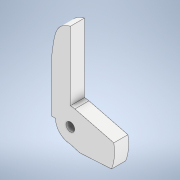
# Autodesk Inventor part: end_cap
Saved by Autodesk Inventor 2022 (Build 260153000, 153)
## iProperties
Created: 2022-12-27
Part Number: end_cap
Material: Типовые
Document SubType Name: Modeling
Designer: akapu
Density: 1 g/cm^3
Appearance: По умолчанию
Author: akapu
Autodesk Inventor part; units mm, degrees
ref_plane "YZ Plane" through (0, 0, 0) normal (1, 0, 0) x (0, 1, 0)
ref_plane "XZ Plane" through (0, 0, 0) normal (0, 1, 0) x (-1, 0, 0)
ref_plane "XY Plane" through (0, 0, 0) normal (0, 0, 1) x (1, 0, 0)
sketch "Эскиз1" plane through (0, 0, 0) normal (0, 0, 1) x (1, 0, 0)
  circle A0 centre (-7, -17) radius 1.5 projected
  line L0 (14, -14.4) -> (14, -5) projected
  arc A1 (14, -5) -> (11, -2) centre (11, -5) ccw projected
  line L1 (11, -2) -> (-7, -2) projected
  line L2 (-7, -2) -> (-7, 15) projected
  line L3 (-14, 9.5) -> (-14, -8.75) projected
  line L4 (-7, -24) -> (7, -24) projected
  arc A2 (7, -24) -> (13.4992, -14.4) centre (7, -17) ccw projected
  line L5 (13.4992, -14.4) -> (14, -14.4) projected
  circle A3 centre (7, -17) radius 2.5 projected
  circle A4 centre (-7, -8.75) radius 5.5 projected
  circle A5 centre (-7, -8.75) radius 6.75 projected
  circle A6 centre (-7, -8.75) radius 5.5 projected
  circle A7 centre (-7, -8.75) radius 16.2607 projected
  circle A8 centre (-7, -8.75) radius 6.75 projected
  circle A9 centre (-7, -8.75) radius 5.5 projected
  arc A10 (46.8183, -61.5099) -> (48.485, -59.5378) centre (46.485, -59.5378) ccw projected
  line L6 (48.485, -59.5378) -> (48.485, -18) projected
  arc A11 (51.485, -15) -> (48.485, -18) centre (51.485, -18) ccw projected
  line L7 (51.485, -15) -> (51.97, -15) projected
  arc A12 (51.97, -15) -> (54.97, -12) centre (51.97, -12) ccw projected
  line L8 (54.97, -5) -> (54.97, -12) projected
  arc A13 (54.97, -5) -> (51.97, -2) centre (51.97, -5) ccw projected
  line L9 (-0.3729, -2) -> (51.97, -2) projected
  arc A14 (-0.3729, -2) -> (-11.03, -11.2398) centre (-0.1714, -12.9982) ccw projected
  line L10 (-11.03, -11.2398) -> (-11.03, -20.501) projected
  arc A15 (-11.03, -20.501) -> (-9.8871, -23.3004) centre (-7.03, -20.501) ccw projected
  arc A16 (-9.03, -25.4) -> (-9.8871, -23.3004) centre (-12.03, -25.4) ccw projected
  line L11 (-9.03, -25.4) -> (-9.03, -104.6) projected
  arc A17 (-9.8871, -106.6996) -> (-9.03, -104.6) centre (-12.03, -104.6) ccw projected
  arc A18 (-9.8871, -106.6996) -> (-11.03, -109.499) centre (-7.03, -109.499) ccw projected
  line L12 (-11.03, -109.499) -> (-11.03, -118.7602) projected
  arc A19 (-11.03, -118.7602) -> (-0.3729, -128) centre (-0.1714, -117.0018) ccw projected
  line L13 (51.97, -128) -> (-0.3729, -128) projected
  arc A20 (51.97, -128) -> (54.97, -125) centre (51.97, -125) ccw projected
  line L14 (54.97, -118) -> (54.97, -125) projected
  arc A21 (54.97, -118) -> (51.97, -115) centre (51.97, -118) ccw projected
  line L15 (51.97, -115) -> (51.485, -115) projected
  arc A22 (48.485, -112) -> (51.485, -115) centre (51.485, -112) ccw projected
  line L16 (48.485, -112) -> (48.485, -80.5022) projected
  arc A23 (48.485, -80.5022) -> (46.8183, -78.5301) centre (46.485, -80.5022) ccw projected
  arc A24 (43.485, -77.3303) -> (46.8183, -78.5301) centre (48.485, -68.67) ccw projected
  arc A25 (42.485, -75.5982) -> (43.485, -77.3303) centre (44.485, -75.5982) ccw projected
  line L17 (42.485, -75.5982) -> (42.485, -64.4418) projected
  arc A26 (43.485, -62.7097) -> (42.485, -64.4418) centre (44.485, -64.4418) ccw projected
  arc A27 (46.8183, -61.5099) -> (43.485, -62.7097) centre (48.485, -71.37) ccw projected
  circle A28 centre (-7, -113) radius 1.5 projected
  circle A29 centre (-7, -17) radius 1.5 projected
  circle A30 centre (48.485, -121.515) radius 1.5 projected
  circle A31 centre (7, -83) radius 1.5 projected
  circle A32 centre (7, -47) radius 1.5 projected
  circle A33 centre (48.485, -8.485) radius 1.5 projected
  circle A34 centre (39.485, -9.27) radius 0.325 projected
  circle A35 centre (38.885, -57.77) radius 0.8 projected
  circle A36 centre (39.385, -64.52) radius 0.5 projected
  circle A37 centre (-5.73, -68.27) radius 0.325 projected
  circle A38 centre (18.2, -105.38) radius 0.325 projected
  circle A39 centre (2.77, -17) radius 0.325 projected
  circle A40 centre (45.185, -81.79) radius 0.325 projected
  circle A41 centre (45.185, -36.51) radius 0.325 projected
  circle A42 centre (2.77, -10) radius 0.325 projected
  circle A43 centre (2.77, -120) radius 0.325 projected
  circle A44 centre (-5.73, -55.42) radius 0.325 projected
  circle A45 centre (29.385, -72.52) radius 0.85 projected
  circle A46 centre (43.885, -57.77) radius 0.8 projected
  circle A47 centre (-1.23, -120) radius 0.325 projected
  circle A48 centre (29.385, -67.52) radius 0.85 projected
  circle A49 centre (18.2, -92.76) radius 0.325 projected
  circle A50 centre (-5.73, -79) radius 0.325 projected
  circle A51 centre (35.215, -122) radius 0.325 projected
  circle A52 centre (33.485, -7.27) radius 0.5 projected
  circle A53 centre (45.185, -101.03) radius 0.325 projected
  circle A54 centre (45.185, -16.27) radius 0.325 projected
  circle A55 centre (35.215, -115) radius 0.325 projected
  circle A56 centre (2.77, -113) radius 0.325 projected
  circle A57 centre (-5.73, -40.84) radius 0.325 projected
  circle A58 centre (39.385, -75.52) radius 0.5 projected
  circle A59 centre (-1.23, -10) radius 0.325 projected
  arc A60 (46.8183, -61.5099) -> (48.485, -59.5378) centre (46.485, -59.5378) ccw projected
  line L18 (48.485, -59.5378) -> (48.485, -18) projected
  arc A61 (51.485, -15) -> (48.485, -18) centre (51.485, -18) ccw projected
  line L19 (51.485, -15) -> (51.97, -15) projected
  arc A62 (51.97, -15) -> (54.97, -12) centre (51.97, -12) ccw projected
  line L20 (54.97, -5) -> (54.97, -12) projected
  arc A63 (54.97, -5) -> (51.97, -2) centre (51.97, -5) ccw projected
  line L21 (-0.3729, -2) -> (51.97, -2) projected
  arc A64 (-0.3729, -2) -> (-11.03, -11.2398) centre (-0.1714, -12.9982) ccw projected
  line L22 (-11.03, -11.2398) -> (-11.03, -20.501) projected
  arc A65 (-11.03, -20.501) -> (-9.8871, -23.3004) centre (-7.03, -20.501) ccw projected
  arc A66 (-9.03, -25.4) -> (-9.8871, -23.3004) centre (-12.03, -25.4) ccw projected
  line L23 (-9.03, -25.4) -> (-9.03, -104.6) projected
  arc A67 (-9.8871, -106.6996) -> (-9.03, -104.6) centre (-12.03, -104.6) ccw projected
  arc A68 (-9.8871, -106.6996) -> (-11.03, -109.499) centre (-7.03, -109.499) ccw projected
  line L24 (-11.03, -109.499) -> (-11.03, -118.7602) projected
  arc A69 (-11.03, -118.7602) -> (-0.3729, -128) centre (-0.1714, -117.0018) ccw projected
  line L25 (51.97, -128) -> (-0.3729, -128) projected
  arc A70 (51.97, -128) -> (54.97, -125) centre (51.97, -125) ccw projected
  line L26 (54.97, -118) -> (54.97, -125) projected
  arc A71 (54.97, -118) -> (51.97, -115) centre (51.97, -118) ccw projected
  line L27 (51.97, -115) -> (51.485, -115) projected
  arc A72 (48.485, -112) -> (51.485, -115) centre (51.485, -112) ccw projected
  line L28 (48.485, -112) -> (48.485, -80.5022) projected
  arc A73 (48.485, -80.5022) -> (46.8183, -78.5301) centre (46.485, -80.5022) ccw projected
  arc A74 (43.485, -77.3303) -> (46.8183, -78.5301) centre (48.485, -68.67) ccw projected
  arc A75 (42.485, -75.5982) -> (43.485, -77.3303) centre (44.485, -75.5982) ccw projected
  line L29 (42.485, -75.5982) -> (42.485, -64.4418) projected
  arc A76 (43.485, -62.7097) -> (42.485, -64.4418) centre (44.485, -64.4418) ccw projected
  arc A77 (46.8183, -61.5099) -> (43.485, -62.7097) centre (48.485, -71.37) ccw projected
  circle A78 centre (-7, -113) radius 1.5 projected
  circle A79 centre (-7, -17) radius 1.5 projected
  circle A80 centre (48.485, -121.515) radius 1.5 projected
  circle A81 centre (7, -83) radius 1.5 projected
  circle A82 centre (7, -47) radius 1.5 projected
  circle A83 centre (48.485, -8.485) radius 1.5 projected
  circle A84 centre (39.485, -9.27) radius 0.325 projected
  circle A85 centre (38.885, -57.77) radius 0.8 projected
  circle A86 centre (39.385, -64.52) radius 0.5 projected
  circle A87 centre (-5.73, -68.27) radius 0.325 projected
  circle A88 centre (18.2, -105.38) radius 0.325 projected
  circle A89 centre (2.77, -17) radius 0.325 projected
  circle A90 centre (45.185, -81.79) radius 0.325 projected
  circle A91 centre (45.185, -36.51) radius 0.325 projected
  circle A92 centre (2.77, -10) radius 0.325 projected
  circle A93 centre (2.77, -120) radius 0.325 projected
  circle A94 centre (-5.73, -55.42) radius 0.325 projected
  circle A95 centre (29.385, -72.52) radius 0.85 projected
  circle A96 centre (43.885, -57.77) radius 0.8 projected
  circle A97 centre (-1.23, -120) radius 0.325 projected
  circle A98 centre (29.385, -67.52) radius 0.85 projected
  circle A99 centre (18.2, -92.76) radius 0.325 projected
  circle A100 centre (-5.73, -79) radius 0.325 projected
  circle A101 centre (35.215, -122) radius 0.325 projected
  circle A102 centre (33.485, -7.27) radius 0.5 projected
  circle A103 centre (45.185, -101.03) radius 0.325 projected
  circle A104 centre (45.185, -16.27) radius 0.325 projected
  circle A105 centre (35.215, -115) radius 0.325 projected
  circle A106 centre (2.77, -113) radius 0.325 projected
  circle A107 centre (-5.73, -40.84) radius 0.325 projected
  circle A108 centre (39.385, -75.52) radius 0.5 projected
  circle A109 centre (-1.23, -10) radius 0.325 projected
  circle A110 centre (-7, -17) radius 1.5 projected
  circle A111 centre (7, -17) radius 2.5 projected
  circle A112 centre (-7, -8.75) radius 16.2607 projected
  arc A113 (46.8183, -61.5099) -> (48.485, -59.5378) centre (46.485, -59.5378) ccw projected
  line L30 (48.485, -59.5378) -> (48.485, -18) projected
  arc A114 (51.485, -15) -> (48.485, -18) centre (51.485, -18) ccw projected
  line L31 (51.485, -15) -> (51.97, -15) projected
  arc A115 (51.97, -15) -> (54.97, -12) centre (51.97, -12) ccw projected
  line L32 (54.97, -5) -> (54.97, -12) projected
  arc A116 (54.97, -5) -> (51.97, -2) centre (51.97, -5) ccw projected
  line L33 (-0.3729, -2) -> (51.97, -2) projected
  arc A117 (-0.3729, -2) -> (-11.03, -11.2398) centre (-0.1714, -12.9982) ccw projected
  line L34 (-11.03, -11.2398) -> (-11.03, -20.501) projected
  arc A118 (-11.03, -20.501) -> (-9.8871, -23.3004) centre (-7.03, -20.501) ccw projected
  arc A119 (-9.03, -25.4) -> (-9.8871, -23.3004) centre (-12.03, -25.4) ccw projected
  line L35 (-9.03, -25.4) -> (-9.03, -104.6) projected
  arc A120 (-9.8871, -106.6996) -> (-9.03, -104.6) centre (-12.03, -104.6) ccw projected
  arc A121 (-9.8871, -106.6996) -> (-11.03, -109.499) centre (-7.03, -109.499) ccw projected
  line L36 (-11.03, -109.499) -> (-11.03, -118.7602) projected
  arc A122 (-11.03, -118.7602) -> (-0.3729, -128) centre (-0.1714, -117.0018) ccw projected
  line L37 (51.97, -128) -> (-0.3729, -128) projected
  arc A123 (51.97, -128) -> (54.97, -125) centre (51.97, -125) ccw projected
  line L38 (54.97, -118) -> (54.97, -125) projected
  arc A124 (54.97, -118) -> (51.97, -115) centre (51.97, -118) ccw projected
  line L39 (51.97, -115) -> (51.485, -115) projected
  arc A125 (48.485, -112) -> (51.485, -115) centre (51.485, -112) ccw projected
  line L40 (48.485, -112) -> (48.485, -80.5022) projected
  arc A126 (48.485, -80.5022) -> (46.8183, -78.5301) centre (46.485, -80.5022) ccw projected
  arc A127 (43.485, -77.3303) -> (46.8183, -78.5301) centre (48.485, -68.67) ccw projected
  arc A128 (42.485, -75.5982) -> (43.485, -77.3303) centre (44.485, -75.5982) ccw projected
  line L41 (42.485, -75.5982) -> (42.485, -64.4418) projected
  arc A129 (43.485, -62.7097) -> (42.485, -64.4418) centre (44.485, -64.4418) ccw projected
  arc A130 (46.8183, -61.5099) -> (43.485, -62.7097) centre (48.485, -71.37) ccw projected
  circle A131 centre (-7, -113) radius 1.5 projected
  circle A132 centre (-7, -17) radius 1.5 projected
  circle A133 centre (48.485, -121.515) radius 1.5 projected
  circle A134 centre (7, -83) radius 1.5 projected
  circle A135 centre (7, -47) radius 1.5 projected
  circle A136 centre (48.485, -8.485) radius 1.5 projected
  circle A137 centre (39.485, -9.27) radius 0.325 projected
  circle A138 centre (38.885, -57.77) radius 0.8 projected
  circle A139 centre (39.385, -64.52) radius 0.5 projected
  circle A140 centre (-5.73, -68.27) radius 0.325 projected
  circle A141 centre (18.2, -105.38) radius 0.325 projected
  circle A142 centre (2.77, -17) radius 0.325 projected
  circle A143 centre (45.185, -81.79) radius 0.325 projected
  circle A144 centre (45.185, -36.51) radius 0.325 projected
  circle A145 centre (2.77, -10) radius 0.325 projected
  circle A146 centre (2.77, -120) radius 0.325 projected
  circle A147 centre (-5.73, -55.42) radius 0.325 projected
  circle A148 centre (29.385, -72.52) radius 0.85 projected
  circle A149 centre (43.885, -57.77) radius 0.8 projected
  circle A150 centre (-1.23, -120) radius 0.325 projected
  circle A151 centre (29.385, -67.52) radius 0.85 projected
  circle A152 centre (18.2, -92.76) radius 0.325 projected
  circle A153 centre (-5.73, -79) radius 0.325 projected
  circle A154 centre (35.215, -122) radius 0.325 projected
  circle A155 centre (33.485, -7.27) radius 0.5 projected
  circle A156 centre (45.185, -101.03) radius 0.325 projected
  circle A157 centre (45.185, -16.27) radius 0.325 projected
  circle A158 centre (35.215, -115) radius 0.325 projected
  circle A159 centre (2.77, -113) radius 0.325 projected
  circle A160 centre (-5.73, -40.84) radius 0.325 projected
  circle A161 centre (39.385, -75.52) radius 0.5 projected
  circle A162 centre (-1.23, -10) radius 0.325 projected
  line L42 (-3.5, -15.3) -> (8.172, -14.6) projected
  line L43 (-1.9964, -14.2379) -> (9.1448, -10.6884) projected
  line L44 (7.4875, -11.5) -> (-3.5, -15.5) projected
  line L45 (-3.5, -15.3) -> (8.172, -14.6) projected
  line L46 (8.172, -14.8) -> (-3.5, -15.5) projected
  arc A163 (8.1929, -15.5) -> (7.4875, -11.5) centre (-3.5, -15.5) ccw projected
  line L47 (-3.5, -15.5) -> (9.3, -15.5) projected
  line L48 (-3.5, -15.5) -> (9.3, -15.5) projected
  circle A164 centre (-7, -17) radius 1.5 projected
  line L49 (14, -14.4) -> (14, -5) projected
  arc A165 (14, -5) -> (11, -2) centre (11, -5) ccw projected
  line L50 (11, -2) -> (-7, -2) projected
  line L51 (-7, -2) -> (-7, 15) projected
  line L52 (-14, 9.5) -> (-14, -8.75) projected
  line L53 (-7, -24) -> (7, -24) projected
  arc A166 (7, -24) -> (13.4992, -14.4) centre (7, -17) ccw projected
  line L54 (13.4992, -14.4) -> (14, -14.4) projected
  circle A167 centre (7, -17) radius 2.5 projected
  circle A168 centre (-7, -17) radius 1.5 projected
  line L55 (14, -14.4) -> (14, -5) projected
  arc A169 (14, -5) -> (11, -2) centre (11, -5) ccw projected
  line L56 (11, -2) -> (-7, -2) projected
  line L57 (-7, -2) -> (-7, 15) projected
  line L58 (-14, 9.5) -> (-14, -8.75) projected
  line L59 (-7, -24) -> (7, -24) projected
  arc A170 (7, -24) -> (13.4992, -14.4) centre (7, -17) ccw projected
  line L60 (13.4992, -14.4) -> (14, -14.4) projected
  circle A171 centre (7, -17) radius 2.5 projected
  line L61 (-3.5, -25.6) -> (-3.5, -15.5) projected
  line L62 (-3.5, -25.6) -> (-3.5, -15.5) projected
  line L63 (-3.5, -15.3) -> (-6.2824, -14.501) projected
  circle A172 centre (-7, -17) radius 2.6 projected
  line L64 (-3.5, -15.5) -> (-7, -15.5) projected
  circle A173 centre (-7, -17) radius 1.5 projected
  line L65 (14, -14.4) -> (14, -5) projected
  arc A174 (14, -5) -> (11, -2) centre (11, -5) ccw projected
  line L66 (11, -2) -> (-7, -2) projected
  line L67 (-7, -2) -> (-7, 15) projected
  line L68 (-14, 9.5) -> (-14, -8.75) projected
  line L69 (-7, -24) -> (7, -24) projected
  arc A175 (7, -24) -> (13.4992, -14.4) centre (7, -17) ccw projected
  line L70 (13.4992, -14.4) -> (14, -14.4) projected
  circle A176 centre (7, -17) radius 2.5 projected
  circle A177 centre (-7, -17) radius 1.5 projected
  circle A178 centre (-7, -17) radius 2.6 projected
  circle A179 centre (-7, -8.75) radius 5.5 projected
  line L71 (-1.9964, -14.2379) -> (-4.8898, -14.1478) projected
  line L72 (-1.9964, -14.2379) -> (9.1448, -10.6884) projected
  line L73 (-1.9964, -14.2379) -> (9.1448, -10.6884) projected
  circle A180 centre (-7, -8.75) radius 6.75 projected
  line L74 (-5.8077, -14.1192) -> (-4.8898, -14.1478) projected
  line L75 (-5.8077, -14.1192) -> (-4.8898, -14.1478) projected
  circle A181 centre (-7, -8.75) radius 5.5 projected
  line L76 (-7, -15.5) -> (-7, -2) projected
  line L77 (-7.1651, -14.2475) -> (-6.2824, -14.501) projected
  line L78 (-3.5, -15.3) -> (-6.2824, -14.501) projected
  circle A182 centre (-7, -17) radius 1.5 projected
  line L79 (14, -14.4) -> (14, -5) projected
  arc A183 (14, -5) -> (11, -2) centre (11, -5) ccw projected
  line L80 (11, -2) -> (-7, -2) projected
  line L81 (-7, -2) -> (-7, 15) projected
  line L82 (-14, 9.5) -> (-14, -8.75) projected
  line L83 (-7, -24) -> (7, -24) projected
  arc A184 (7, -24) -> (13.4992, -14.4) centre (7, -17) ccw projected
  line L84 (13.4992, -14.4) -> (14, -14.4) projected
  circle A185 centre (7, -17) radius 2.5 projected
  circle A186 centre (-7, -17) radius 2.6 projected
  circle A187 centre (-7, -17) radius 2.6 projected
  line L85 (-7, -15.5) -> (-7, -2) projected
  circle A188 centre (-7, -17) radius 1.5 projected
  line L86 (14, -14.4) -> (14, -5) projected
  arc A189 (14, -5) -> (11, -2) centre (11, -5) ccw projected
  line L87 (11, -2) -> (-7, -2) projected
  line L88 (-7, -2) -> (-7, 15) projected
  line L89 (-14, 9.5) -> (-14, -8.75) projected
  line L90 (-7, -24) -> (7, -24) projected
  arc A190 (7, -24) -> (13.4992, -14.4) centre (7, -17) ccw projected
  line L91 (13.4992, -14.4) -> (14, -14.4) projected
  circle A191 centre (7, -17) radius 2.5 projected
  circle A192 centre (-7, -17) radius 1.5 projected
  line L92 (14, -14.4) -> (14, -5) projected
  arc A193 (14, -5) -> (11, -2) centre (11, -5) ccw projected
  line L93 (11, -2) -> (-7, -2) projected
  line L94 (-7, -2) -> (-7, 15) projected
  line L95 (-14, 9.5) -> (-14, -8.75) projected
  line L96 (-7, -24) -> (7, -24) projected
  arc A194 (7, -24) -> (13.4992, -14.4) centre (7, -17) ccw projected
  line L97 (13.4992, -14.4) -> (14, -14.4) projected
  circle A195 centre (7, -17) radius 2.5 projected
  circle A196 centre (-7, -8.75) radius 5.5 projected
  circle A197 centre (-7, -17) radius 1.5 projected
  line L98 (14, -14.4) -> (14, -5) projected
  arc A198 (14, -5) -> (11, -2) centre (11, -5) ccw projected
  line L99 (11, -2) -> (-7, -2) projected
  line L100 (-7, -2) -> (-7, 15) projected
  line L101 (-14, 9.5) -> (-14, -8.75) projected
  line L102 (-7, -24) -> (7, -24) projected
  arc A199 (7, -24) -> (13.4992, -14.4) centre (7, -17) ccw projected
  line L103 (13.4992, -14.4) -> (14, -14.4) projected
  circle A200 centre (7, -17) radius 2.5 projected
  circle A201 centre (-7, -8.75) radius 1.6 projected
  circle A202 centre (-7, -8.75) radius 1.6 projected
  line L104 (-7, -15.5) -> (-7, -2) projected
  circle A203 centre (-7, -17) radius 1.5 projected
  line L105 (14, -14.4) -> (14, -5) projected
  arc A204 (14, -5) -> (11, -2) centre (11, -5) ccw projected
  line L106 (11, -2) -> (-7, -2) projected
  line L107 (-7, -2) -> (-7, 15) projected
  line L108 (-14, 9.5) -> (-14, -8.75) projected
  line L109 (-7, -24) -> (7, -24) projected
  arc A205 (7, -24) -> (13.4992, -14.4) centre (7, -17) ccw projected
  line L110 (13.4992, -14.4) -> (14, -14.4) projected
  circle A206 centre (7, -17) radius 2.5 projected
  circle A207 centre (-7, -17) radius 1.5 projected
  line L111 (14, -14.4) -> (14, -5) projected
  arc A208 (14, -5) -> (11, -2) centre (11, -5) ccw projected
  line L112 (11, -2) -> (-7, -2) projected
  line L113 (-7, -2) -> (-7, 15) projected
  line L114 (-14, 9.5) -> (-14, -8.75) projected
  line L115 (-7, -24) -> (7, -24) projected
  arc A209 (7, -24) -> (13.4992, -14.4) centre (7, -17) ccw projected
  line L116 (13.4992, -14.4) -> (14, -14.4) projected
  circle A210 centre (7, -17) radius 2.5 projected
  line L117 (-7, -8.75) -> (8.9993, -5.8462) projected
  circle A211 centre (-7, -17) radius 1.5 projected
  line L118 (14, -14.4) -> (14, -5) projected
  arc A212 (14, -5) -> (11, -2) centre (11, -5) ccw projected
  line L119 (11, -2) -> (-7, -2) projected
  line L120 (-7, -2) -> (-7, 15) projected
  line L121 (-14, 9.5) -> (-14, -8.75) projected
  line L122 (-7, -24) -> (7, -24) projected
  arc A213 (7, -24) -> (13.4992, -14.4) centre (7, -17) ccw projected
  line L123 (13.4992, -14.4) -> (14, -14.4) projected
  circle A214 centre (7, -17) radius 2.5 projected
  line L124 (7.7935, -2) -> (-7, -8.75) projected
  line L125 (7.7935, -2) -> (-7, -8.75) projected
  circle A215 centre (-7, -17) radius 1.5 projected
  line L126 (14, -14.4) -> (14, -5) projected
  arc A216 (14, -5) -> (11, -2) centre (11, -5) ccw projected
  line L127 (11, -2) -> (-7, -2) projected
  line L128 (-7, -2) -> (-7, 15) projected
  line L129 (-14, 9.5) -> (-14, -8.75) projected
  line L130 (-7, -24) -> (7, -24) projected
  arc A217 (7, -24) -> (13.4992, -14.4) centre (7, -17) ccw projected
  line L131 (13.4992, -14.4) -> (14, -14.4) projected
  circle A218 centre (7, -17) radius 2.5 projected
  circle A219 centre (-7, -8.75) radius 6.75 projected
  circle A220 centre (-7, -17) radius 1.5 projected
  line L132 (14, -14.4) -> (14, -5) projected
  arc A221 (14, -5) -> (11, -2) centre (11, -5) ccw projected
  line L133 (11, -2) -> (-7, -2) projected
  line L134 (-7, -2) -> (-7, 15) projected
  line L135 (-14, 9.5) -> (-14, -8.75) projected
  line L136 (-7, -24) -> (7, -24) projected
  arc A222 (7, -24) -> (13.4992, -14.4) centre (7, -17) ccw projected
  line L137 (13.4992, -14.4) -> (14, -14.4) projected
  circle A223 centre (7, -17) radius 2.5 projected
  circle A224 centre (-7, -8.75) radius 6.75 projected
  circle A225 centre (-7, -17) radius 2.6 projected
  circle A226 centre (-7, -17) radius 2.6 projected
  circle A227 centre (-7, -17) radius 1.5 projected
  line L138 (14, -14.4) -> (14, -5) projected
  arc A228 (14, -5) -> (11, -2) centre (11, -5) ccw projected
  line L139 (11, -2) -> (-7, -2) projected
  line L140 (-7, -2) -> (-7, 15) projected
  line L141 (-14, 9.5) -> (-14, -8.75) projected
  line L142 (-7, -24) -> (7, -24) projected
  arc A229 (7, -24) -> (13.4992, -14.4) centre (7, -17) ccw projected
  line L143 (13.4992, -14.4) -> (14, -14.4) projected
  circle A230 centre (7, -17) radius 2.5 projected
  line L144 (8.9993, -5.8462) -> (-1.6265, -3.1497) projected
  line L145 (8.9993, -5.8462) -> (-1.6265, -3.1497) projected
  circle A231 centre (-7, -17) radius 1.5 projected
  line L146 (14, -14.4) -> (14, -5) projected
  arc A232 (14, -5) -> (11, -2) centre (11, -5) ccw projected
  line L147 (11, -2) -> (-7, -2) projected
  line L148 (-7, -2) -> (-7, 15) projected
  line L149 (-14, 9.5) -> (-14, -8.75) projected
  line L150 (-7, -24) -> (7, -24) projected
  arc A233 (7, -24) -> (13.4992, -14.4) centre (7, -17) ccw projected
  line L151 (13.4992, -14.4) -> (14, -14.4) projected
  circle A234 centre (7, -17) radius 2.5 projected
  circle A235 centre (-7, -17) radius 1.5 projected
  line L152 (14, -14.4) -> (14, -5) projected
  arc A236 (14, -5) -> (11, -2) centre (11, -5) ccw projected
  line L153 (11, -2) -> (-7, -2) projected
  line L154 (-7, -2) -> (-7, 15) projected
  line L155 (-14, 9.5) -> (-14, -8.75) projected
  line L156 (-7, -24) -> (7, -24) projected
  arc A237 (7, -24) -> (13.4992, -14.4) centre (7, -17) ccw projected
  line L157 (13.4992, -14.4) -> (14, -14.4) projected
  circle A238 centre (7, -17) radius 2.5 projected
  circle A239 centre (-7, -17) radius 1.5 projected
  line L158 (14, -14.4) -> (14, -5) projected
  arc A240 (14, -5) -> (11, -2) centre (11, -5) ccw projected
  line L159 (11, -2) -> (-7, -2) projected
  line L160 (-7, -2) -> (-7, 15) projected
  line L161 (-14, 9.5) -> (-14, -8.75) projected
  line L162 (-7, -24) -> (7, -24) projected
  arc A241 (7, -24) -> (13.4992, -14.4) centre (7, -17) ccw projected
  line L163 (13.4992, -14.4) -> (14, -14.4) projected
  circle A242 centre (7, -17) radius 2.5 projected
  circle A243 centre (-7, -8.75) radius 6.75 projected
  line L164 (11, -2) -> (-7, -2) projected
  circle A244 centre (-7, -17) radius 1.5 projected
  line L165 (14, -14.4) -> (14, -5) projected
  arc A245 (14, -5) -> (11, -2) centre (11, -5) ccw projected
  line L166 (11, -2) -> (-7, -2) projected
  line L167 (-7, -2) -> (-7, 15) projected
  line L168 (-14, 9.5) -> (-14, -8.75) projected
  line L169 (-7, -24) -> (7, -24) projected
  arc A246 (7, -24) -> (13.4992, -14.4) centre (7, -17) ccw projected
  line L170 (13.4992, -14.4) -> (14, -14.4) projected
  circle A247 centre (7, -17) radius 2.5 projected
  line L171 (-7, 15) -> (-7, 23.3611) projected
  line L172 (8.9993, -5.8462) -> (-1.6265, -3.1497) projected
  line L173 (8.9993, -5.8462) -> (-6.1569, -2) projected
  line L174 (8.9993, -5.8462) -> (-1.6265, -3.1497) projected
  line L175 (8.9993, -5.8462) -> (-6.1569, -2) projected
  line L176 (-14, -8.75) -> (-14, -3.75)
  line L177 (-14, -8.75) -> (-12.5, -8.75)
  spline S0 degree 3 poles (-7, 23.3611) (-12.8051, 21.7936) (-12.8999, 17.7118) (-14, 9.5) knots -0.659309 -0.659309 -0.659309 -0.659309 0 0 0 0 projected
  line L178 (-14, -8.75) -> (-12.7, -8.75) projected
  arc A248 (-12.7, -8.75) -> (-11.9767, -11.529) centre (-7, -8.75) ccw projected
  line L179 (-11.9767, -11.529) -> (-9.4156, -17.9617) projected
  arc A249 (-9.4156, -17.9617) -> (-7, -19.6) centre (-7, -17) ccw projected
  arc A250 (-7, -24) -> (-7, -19.6) centre (-7, -21.8) ccw projected
  line L180 (-7, 15) -> (-7, 23.3611) projected
  spline S1 degree 3 poles (-7, 23.3611) (-12.8051, 21.7936) (-12.8999, 17.7118) (-14, 9.5) knots -0.659309 -0.659309 -0.659309 -0.659309 0 0 0 0 projected
  line L181 (-14, -8.75) -> (-12.7, -8.75) projected
  arc A251 (-12.7, -8.75) -> (-11.9767, -11.529) centre (-7, -8.75) ccw projected
  line L182 (-11.9767, -11.529) -> (-9.4156, -17.9617) projected
  arc A252 (-9.4156, -17.9617) -> (-7, -19.6) centre (-7, -17) ccw projected
  arc A253 (-7, -24) -> (-7, -19.6) centre (-7, -21.8) ccw projected
  line L183 (-7, 15) -> (-7, 23.3611) projected
  spline S2 degree 3 poles (-7, 23.3611) (-12.8051, 21.7936) (-12.8999, 17.7118) (-14, 9.5) knots -0.659309 -0.659309 -0.659309 -0.659309 0 0 0 0 projected
  line L184 (-14, -8.75) -> (-12.7, -8.75) projected
  arc A254 (-12.7, -8.75) -> (-11.9767, -11.529) centre (-7, -8.75) ccw projected
  line L185 (-11.9767, -11.529) -> (-9.4156, -17.9617) projected
  arc A255 (-9.4156, -17.9617) -> (-7, -19.6) centre (-7, -17) ccw projected
  arc A256 (-7, -24) -> (-7, -19.6) centre (-7, -21.8) ccw projected
  line L186 (-7, 15) -> (-7, 23.3611) projected
  spline S3 degree 3 poles (-7, 23.3611) (-12.8051, 21.7936) (-12.8999, 17.7118) (-14, 9.5) knots -0.659309 -0.659309 -0.659309 -0.659309 0 0 0 0 projected
  line L187 (-14, -8.75) -> (-12.7, -8.75) projected
  arc A257 (-12.7, -8.75) -> (-11.9767, -11.529) centre (-7, -8.75) ccw projected
  line L188 (-11.9767, -11.529) -> (-9.4156, -17.9617) projected
  arc A258 (-9.4156, -17.9617) -> (-7, -19.6) centre (-7, -17) ccw projected
  arc A259 (-7, -24) -> (-7, -19.6) centre (-7, -21.8) ccw projected
  line L189 (-7, 15) -> (-7, 23.3611) projected
  spline S4 degree 3 poles (-7, 23.3611) (-12.8051, 21.7936) (-12.8999, 17.7118) (-14, 9.5) knots -0.659309 -0.659309 -0.659309 -0.659309 0 0 0 0 projected
  line L190 (-14, -8.75) -> (-12.7, -8.75) projected
  arc A260 (-12.7, -8.75) -> (-11.9767, -11.529) centre (-7, -8.75) ccw projected
  line L191 (-11.9767, -11.529) -> (-9.4156, -17.9617) projected
  arc A261 (-9.4156, -17.9617) -> (-7, -19.6) centre (-7, -17) ccw projected
  arc A262 (-7, -24) -> (-7, -19.6) centre (-7, -21.8) ccw projected
  line L192 (-7, 15) -> (-7, 23.3611) projected
  spline S5 degree 3 poles (-7, 23.3611) (-12.8051, 21.7936) (-12.8999, 17.7118) (-14, 9.5) knots -0.659309 -0.659309 -0.659309 -0.659309 0 0 0 0 projected
  line L193 (-14, -8.75) -> (-12.7, -8.75) projected
  arc A263 (-12.7, -8.75) -> (-11.9767, -11.529) centre (-7, -8.75) ccw projected
  line L194 (-11.9767, -11.529) -> (-9.4156, -17.9617) projected
  arc A264 (-9.4156, -17.9617) -> (-7, -19.6) centre (-7, -17) ccw projected
  arc A265 (-7, -24) -> (-7, -19.6) centre (-7, -21.8) ccw projected
  line L195 (-7, 15) -> (-7, 23.3611) projected
  spline S6 degree 3 poles (-7, 23.3611) (-12.8051, 21.7936) (-12.8999, 17.7118) (-14, 9.5) knots -0.659309 -0.659309 -0.659309 -0.659309 0 0 0 0 projected
  line L196 (-14, -8.75) -> (-12.7, -8.75) projected
  arc A266 (-12.7, -8.75) -> (-11.9767, -11.529) centre (-7, -8.75) ccw projected
  line L197 (-11.9767, -11.529) -> (-9.4156, -17.9617) projected
  arc A267 (-9.4156, -17.9617) -> (-7, -19.6) centre (-7, -17) ccw projected
  arc A268 (-7, -24) -> (-7, -19.6) centre (-7, -21.8) ccw projected
  line L198 (-7, 15) -> (-7, 23.3611) projected
  spline S7 degree 3 poles (-7, 23.3611) (-12.8051, 21.7936) (-12.8999, 17.7118) (-14, 9.5) knots -0.659309 -0.659309 -0.659309 -0.659309 0 0 0 0 projected
  line L199 (-14, -8.75) -> (-12.7, -8.75) projected
  arc A269 (-12.7, -8.75) -> (-11.9767, -11.529) centre (-7, -8.75) ccw projected
  line L200 (-11.9767, -11.529) -> (-9.4156, -17.9617) projected
  arc A270 (-9.4156, -17.9617) -> (-7, -19.6) centre (-7, -17) ccw projected
  arc A271 (-7, -24) -> (-7, -19.6) centre (-7, -21.8) ccw projected
  line L201 (-7, 15) -> (-7, 23.3611) projected
  spline S8 degree 3 poles (-7, 23.3611) (-12.8051, 21.7936) (-12.8999, 17.7118) (-14, 9.5) knots -0.659309 -0.659309 -0.659309 -0.659309 0 0 0 0 projected
  line L202 (-14, -8.75) -> (-12.7, -8.75) projected
  arc A272 (-12.7, -8.75) -> (-11.9767, -11.529) centre (-7, -8.75) ccw projected
  line L203 (-11.9767, -11.529) -> (-9.4156, -17.9617) projected
  arc A273 (-9.4156, -17.9617) -> (-7, -19.6) centre (-7, -17) ccw projected
  arc A274 (-7, -24) -> (-7, -19.6) centre (-7, -21.8) ccw projected
  line L204 (-7, 15) -> (-7, 23.3611) projected
  spline S9 degree 3 poles (-7, 23.3611) (-12.8051, 21.7936) (-12.8999, 17.7118) (-14, 9.5) knots -0.659309 -0.659309 -0.659309 -0.659309 0 0 0 0 projected
  line L205 (-14, -8.75) -> (-12.7, -8.75) projected
  arc A275 (-12.7, -8.75) -> (-11.9767, -11.529) centre (-7, -8.75) ccw projected
  line L206 (-11.9767, -11.529) -> (-9.4156, -17.9617) projected
  arc A276 (-9.4156, -17.9617) -> (-7, -19.6) centre (-7, -17) ccw projected
  arc A277 (-7, -24) -> (-7, -19.6) centre (-7, -21.8) ccw projected
  line L207 (-7, 15) -> (-7, 23.3611) projected
  spline S10 degree 3 poles (-7, 23.3611) (-12.8051, 21.7936) (-12.8999, 17.7118) (-14, 9.5) knots -0.659309 -0.659309 -0.659309 -0.659309 0 0 0 0 projected
  line L208 (-14, -8.75) -> (-12.7, -8.75) projected
  arc A278 (-12.7, -8.75) -> (-11.9767, -11.529) centre (-7, -8.75) ccw projected
  line L209 (-11.9767, -11.529) -> (-9.4156, -17.9617) projected
  arc A279 (-9.4156, -17.9617) -> (-7, -19.6) centre (-7, -17) ccw projected
  arc A280 (-7, -24) -> (-7, -19.6) centre (-7, -21.8) ccw projected
  line L210 (-7, 15) -> (-7, 23.3611) projected
  spline S11 degree 3 poles (-7, 23.3611) (-12.8051, 21.7936) (-12.8999, 17.7118) (-14, 9.5) knots -0.659309 -0.659309 -0.659309 -0.659309 0 0 0 0 projected
  line L211 (-14, -8.75) -> (-12.7, -8.75) projected
  arc A281 (-12.7, -8.75) -> (-11.9767, -11.529) centre (-7, -8.75) ccw projected
  line L212 (-11.9767, -11.529) -> (-9.4156, -17.9617) projected
  arc A282 (-9.4156, -17.9617) -> (-7, -19.6) centre (-7, -17) ccw projected
  arc A283 (-7, -24) -> (-7, -19.6) centre (-7, -21.8) ccw projected
  line L213 (-7, 15) -> (-7, 23.3611) projected
  spline S12 degree 3 poles (-7, 23.3611) (-12.8051, 21.7936) (-12.8999, 17.7118) (-14, 9.5) knots -0.659309 -0.659309 -0.659309 -0.659309 0 0 0 0 projected
  line L214 (-14, -8.75) -> (-12.7, -8.75) projected
  arc A284 (-12.7, -8.75) -> (-11.9767, -11.529) centre (-7, -8.75) ccw projected
  line L215 (-11.9767, -11.529) -> (-9.4156, -17.9617) projected
  arc A285 (-9.4156, -17.9617) -> (-7, -19.6) centre (-7, -17) ccw projected
  arc A286 (-7, -24) -> (-7, -19.6) centre (-7, -21.8) ccw projected
  line L216 (-7, 15) -> (-7, 23.3611) projected
  spline S13 degree 3 poles (-7, 23.3611) (-12.8051, 21.7936) (-12.8999, 17.7118) (-14, 9.5) knots -0.659309 -0.659309 -0.659309 -0.659309 0 0 0 0 projected
  line L217 (-14, -8.75) -> (-12.7, -8.75) projected
  arc A287 (-12.7, -8.75) -> (-11.9767, -11.529) centre (-7, -8.75) ccw projected
  line L218 (-11.9767, -11.529) -> (-9.4156, -17.9617) projected
  arc A288 (-9.4156, -17.9617) -> (-7, -19.6) centre (-7, -17) ccw projected
  arc A289 (-7, -24) -> (-7, -19.6) centre (-7, -21.8) ccw projected
  line L219 (-7, 15) -> (-7, 23.3611) projected
  spline S14 degree 3 poles (-7, 23.3611) (-12.8051, 21.7936) (-12.8999, 17.7118) (-14, 9.5) knots -0.659309 -0.659309 -0.659309 -0.659309 0 0 0 0 projected
  line L220 (-14, -8.75) -> (-12.7, -8.75) projected
  arc A290 (-12.7, -8.75) -> (-11.9767, -11.529) centre (-7, -8.75) ccw projected
  line L221 (-11.9767, -11.529) -> (-9.4156, -17.9617) projected
  arc A291 (-9.4156, -17.9617) -> (-7, -19.6) centre (-7, -17) ccw projected
  arc A292 (-7, -24) -> (-7, -19.6) centre (-7, -21.8) ccw projected
  line L222 (-7, 15) -> (-7, 23.3611) projected
  spline S15 degree 3 poles (-7, 23.3611) (-12.8051, 21.7936) (-12.8999, 17.7118) (-14, 9.5) knots -0.659309 -0.659309 -0.659309 -0.659309 0 0 0 0 projected
  line L223 (-14, -8.75) -> (-12.7, -8.75) projected
  arc A293 (-12.7, -8.75) -> (-11.9767, -11.529) centre (-7, -8.75) ccw projected
  line L224 (-11.9767, -11.529) -> (-9.4156, -17.9617) projected
  arc A294 (-9.4156, -17.9617) -> (-7, -19.6) centre (-7, -17) ccw projected
  arc A295 (-7, -24) -> (-7, -19.6) centre (-7, -21.8) ccw projected
  line L225 (-7, 15) -> (-7, 23.3611) projected
  spline S16 degree 3 poles (-7, 23.3611) (-12.8051, 21.7936) (-12.8999, 17.7118) (-14, 9.5) knots -0.659309 -0.659309 -0.659309 -0.659309 0 0 0 0 projected
  line L226 (-14, -8.75) -> (-12.7, -8.75) projected
  arc A296 (-12.7, -8.75) -> (-11.9767, -11.529) centre (-7, -8.75) ccw projected
  line L227 (-11.9767, -11.529) -> (-9.4156, -17.9617) projected
  arc A297 (-9.4156, -17.9617) -> (-7, -19.6) centre (-7, -17) ccw projected
  arc A298 (-7, -24) -> (-7, -19.6) centre (-7, -21.8) ccw projected
  line L228 (-7, 15) -> (-7, 23.3611) projected
  spline S17 degree 3 poles (-7, 23.3611) (-12.8051, 21.7936) (-12.8999, 17.7118) (-14, 9.5) knots -0.659309 -0.659309 -0.659309 -0.659309 0 0 0 0 projected
  line L229 (-14, -8.75) -> (-12.7, -8.75) projected
  arc A299 (-12.7, -8.75) -> (-11.9767, -11.529) centre (-7, -8.75) ccw projected
  line L230 (-11.9767, -11.529) -> (-9.4156, -17.9617) projected
  arc A300 (-9.4156, -17.9617) -> (-7, -19.6) centre (-7, -17) ccw projected
  arc A301 (-7, -24) -> (-7, -19.6) centre (-7, -21.8) ccw projected
  line L231 (-7, 15) -> (-7, 23.3611) projected
  point P0 (0, 0)
  point P1 (-4, 18)
  point P2 (2, 24)
  point P3 (-2.9442, 24)
  point P4 (-14, -17)
  point P5 (-5.5, -17)
  point P6 (-5.3397, -2.2074)
  point P7 (-7, -14.2949)
  point P8 (-7, -14.25)
  dimension "d0" = 5
  constraints: 8 horizontal alignment, 2 vertical, 1 coincident, 1 end point, 1 point on circle, 145 other
extrude "Выдавливание1" add sketch "Эскиз1" along normal blind 5.2 contours L63 L77 L76 A4 L74 L71 A5 | A5 L71 L43 A7 L42 A163 L44 L63 | L71 L74 A4 L117 A5 | A5 L117 A7 L43 L71 | L44 A163 L42 A3 | L76 A201 L117 A4 | A4 L10 A14 L76 A201 | L177 L3 A7 L2 A5 | A5 L76 A4 L177 | A4 L76 A14 L10 | A3 L42 | A5 A14 A4 L76 | L117 A4 L124 A5 | A5 L124 L144 L117 | L76 A14 A4 L124 A201 | A7 L3 S0 L171 L2 | L173 A14 A5 | A4 A14 L76 | L124 A4 A14 A5 | A5 A14 L173 L144 L124 | L117 A201 L124 A4 | A42 | A59
